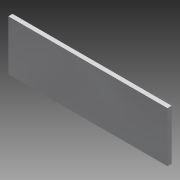
# Autodesk Inventor part: DishFront_BackPlate_Blank
Saved by Autodesk Inventor 2014 (Build 180170000, 170)
## iProperties
Created: 2015-01-07
Part Number: DishFront_BackPlate_Blank
Material: Generic
Document SubType Name: Modeling
Designer: Owner
Density: 1 g/cm^3
Appearance: Aluminum - Polished
Author: Owner
Autodesk Inventor part; units mm, degrees
ref_plane "YZ Plane" through (0, 0, 0) normal (1, 0, 0) x (0, 1, 0)
ref_plane "XZ Plane" through (0, 0, 0) normal (0, 1, 0) x (-1, 0, 0)
ref_plane "XY Plane" through (0, 0, 0) normal (0, 0, 1) x (1, 0, 0)
sketch "Sketch1" plane through (0, 0, 0) normal (0, 0, 1) x (1, 0, 0)
  line L0 (-131.3923, -13.6452) -> (-10.7423, -13.6452)
  line L1 (-10.7423, -13.6452) -> (-10.7423, -51.7452)
  line L2 (-10.7423, -51.7452) -> (-131.3923, -51.7452)
  line L3 (-131.3923, -51.7452) -> (-131.3923, -13.6452)
  point P0 (0, 0)
  dimension "d0" = 120.65
  dimension "d1" = 38.1
  constraints: 8 end point, 2 parallel, 1 horizontal, 1 perpendicular
  measures "d0" distance of L0.start L0.end
  measures "d1" distance of L0.end L1.end
extrude "Extrusion1" add sketch "Sketch1" along normal blind 3.175
body "Solid1"
